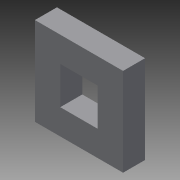
# Autodesk Inventor part: SquareHoleCalibration
Saved by Autodesk Inventor 2015 (Build 190159000, 159)
## iProperties
Created: 2015-04-21
Part Number: SquareHoleCalibration
Material: Generic
Document SubType Name: Modeling
Designer: doctor
Density: 1 g/cm^3
Appearance: Default
Author: doctor
Autodesk Inventor part; units mm, degrees
ref_plane "YZ Plane" through (0, 0, 0) normal (1, 0, 0) x (0, 1, 0)
ref_plane "XZ Plane" through (0, 0, 0) normal (0, 1, 0) x (-1, 0, 0)
ref_plane "XY Plane" through (0, 0, 0) normal (0, 0, 1) x (1, 0, 0)
sketch "Sketch1" plane through (0, 0, 0) normal (0, 1, 0) x (-1, 0, 0)
  line L0 (0, 0) -> (20, 0)
  line L1 (20, 0) -> (20, -20)
  line L2 (20, -20) -> (0, -20)
  line L3 (0, -20) -> (0, 0)
  line L4 (14.25, -5.75) -> (5.75, -5.75)
  line L5 (5.75, -5.75) -> (5.75, -14.25)
  line L6 (5.75, -14.25) -> (14.25, -14.25)
  line L7 (14.25, -14.25) -> (14.25, -5.75)
  line L8 (20, -20) -> (0, 0) construction
  line L9 (14.25, -5.75) -> (5.75, -14.25) construction
  point P0 (10, -10)
  dimension "d0" = 20
  dimension "d1" = 20
  dimension "d2" = 8.5
  dimension "d3" = 8.5
  constraints: 20 end point, 4 parallel, 2 horizontal, 2 midpoint, 2 perpendicular
  measures "d0" distance of L1.end L2.end
  measures "d1" distance of L0.end L1.end
  measures "d2" distance of L6.end L5.end
  measures "d3" distance of L5.end L4.end
extrude "Extrusion1" add sketch "Sketch1" along normal blind 5
body "Solid1"
